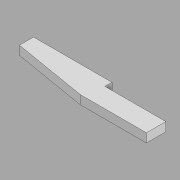
# Autodesk Inventor part: 102.001.02_Anbindung_Vereinzelung
Saved by Autodesk Inventor 2021 (Build 250183000, 183)
## iProperties
Created: 2021-11-26
Part Number: 102.001.02_Anbindung_Vereinzelung
Material: Generisch
Document SubType Name: Modeling
Designer: Oliver Ungerer
Density: 1 g/cm^3
Appearance: Vorgabe
Author: Oliver Ungerer
Autodesk Inventor part; units mm, degrees
ref_plane "YZ Plane" through (0, 0, 0) normal (1, 0, 0) x (0, 1, 0)
ref_plane "XZ Plane" through (0, 0, 0) normal (0, 1, 0) x (-1, 0, 0)
ref_plane "XY Plane" through (0, 0, 0) normal (0, 0, 1) x (1, 0, 0)
sketch "Skizze6" plane through (0, 0, 0) normal (0, 1, 0) x (-1, 0, 0)
  line L0 (69, 0) -> (158, 0)
  line L1 (158, 0) -> (158, 16)
  line L2 (0, 30) -> (0, 8)
  line L3 (0, 8) -> (69, 8)
  line L4 (69, 8) -> (69, 0)
  line L5 (0, 30) -> (75, 30)
  line L6 (75, 30) -> (158, 16)
  point P0 (0, 0)
  dimension "d34" = 89
  dimension "d35" = 22
  dimension "d36" = 30
  dimension "d37" = 158
  dimension "d38" = 75
  dimension "d41" = 16
  constraints: 14 end point, 3 perpendicular, 2 horizontal, 2 point on line, 1 parallel
  measures "d34" distance between parallel lines of L4 L1
  measures "d35" distance from line of L2.start L3
  measures "d36" distance from line of L5 point (0, 0)
  measures "d37" distance from line of point (0, 0) L1
  measures "d38" distance of L2.start L5.end
  measures "d41" distance of L0.end L1.end
extrude "Extrusion2" add sketch "Skizze6" along normal blind 10
